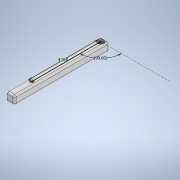
# Autodesk Inventor part: spincoater dispense arm
Saved by Autodesk Inventor 2020 (Build 240168000, 168)
## iProperties
Created: 2023-05-01
Part Number: spincoater dispense arm
Material: Generic
Document SubType Name: Modeling
Designer: Beaucage
Density: 1 g/cm^3
Appearance: Default
Author: Beaucage
Autodesk Inventor part; units mm, degrees
ref_plane "YZ Plane" through (0, 0, 0) normal (1, 0, 0) x (0, 1, 0)
ref_plane "XZ Plane" through (0, 0, 0) normal (0, 1, 0) x (-1, 0, 0)
ref_plane "XY Plane" through (0, 0, 0) normal (0, 0, 1) x (1, 0, 0)
sketch "Sketch1" plane through (0, 0, 0) normal (0, 1, 0) x (-1, 0, 0)
  line L0 (-6.35, 6.35) -> (6.35, 6.35)
  line L1 (6.35, 6.35) -> (6.35, -6.35)
  line L2 (6.35, -6.35) -> (-6.35, -6.35)
  line L3 (-6.35, -6.35) -> (-6.35, 6.35)
  line L4 (-6.35, 6.35) -> (6.35, -6.35) construction
  line L5 (6.35, 6.35) -> (-6.35, -6.35) construction
  circle A0 centre (0, 0) radius 4.7625
  dimension "d0" = 12.7
  dimension "d1" = 12.7
  dimension "d2" = 9.525
  constraints: 12 end point, 2 midpoint, 2 parallel, 1 centre point, 1 coincident, 1 horizontal, 1 perpendicular
  measures "d0" distance of L1.end L2.end
  measures "d1" distance of L0.end L1.end
  measures "d2" diameter of A0
extrude "Extrusion1" add sketch "Sketch1" along normal blind 12.7
sketch "Sketch2" plane through (-6.35, 0, 6.35) normal (0, 0, 1) x (1, 0, 0)
  line L0 (6.35, 0) -> (6.35, 6.35)
  circle A0 centre (6.35, 6.35) radius 1.5875
  dimension "d5" = 6.35
  dimension "d6" = 3.175
  constraints: 2 end point, 1 centre point, 1 coincident, 1 vertical
  measures "d5" distance of L0.start L0.end
  measures "d6" diameter of A0
extrude "Extrusion2" add sketch "Sketch2" against normal blind 4.445
sketch "Sketch3" plane through (-6.35, 0, 6.35) normal (0, 0, 1) x (1, 0, 0)
  line L0 (12.7, 0) -> (0, 0) projected
  line L1 (12.7, 0) -> (12.7, 12.7) projected
  line L2 (0, 0) -> (12.7, 0)
  line L3 (12.7, 0) -> (12.7, 12.7)
  line L4 (12.7, 12.7) -> (0, 12.7)
  line L5 (0, 12.7) -> (0, 0)
  point P0 (6.35, 0)
  constraints: 8 end point, 2 parallel, 1 horizontal, 1 perpendicular
extrude "Extrusion3" add sketch "Sketch3" along normal blind 127
fillet "Fillet1" radius 2.54 12 edges at (6.35, 12.7, 63.5) (6.35, 0, 63.5) (-6.35, 12.7, 63.5) (-6.35, 0, 63.5) (-6.35, 6.35, 133.35) (0, 0, 133.35) (6.35, 6.35, 133.35) (0, 12.7, 133.35) (-6.35, 6.35, -6.35) (6.35, 6.35, -6.35) (0, 12.7, -6.35) (0, 0, -6.35)
sketch "Sketch4" plane through (0, 12.7, 0) normal (0, 1, 0) x (1, 0, 0)
  line L0 (0, 0) -> (0, -101.854)
  line L1 (0, 0) -> (101.854, 0) construction
  dimension "d12" = 101.854
  dimension "d13" = 90
  constraints: 4 end point, 1 horizontal, 1 perpendicular, 1 vertical
  measures "d12" distance of L0.start L0.end
  measures "d13" angle of L0 L1
hole "Hole1" at (0, 12.7, 101.854) direction (0, -1, 0) diameter 5.4102 depth 6.35
hole "Hole2" at (0, 12.7, 101.854) direction (0, -1, 0) diameter 3.175 depth 25.4 tip angle 118
sketch "Sketch5" plane through (-6.35, 2.54, -3.81) normal (-1, 0, 0) x (0, 0, 1)
  line L0 (3.81, -2.54) -> (96.774, -2.54)
  line L1 (3.81, -2.54) -> (96.774, -2.54) construction
  line L2 (96.774, -2.54) -> (96.774, 3.81)
  line L3 (134.62, 0) -> (0, 0) projected
  line L4 (96.774, -2.54) -> (103.124, -2.54) construction
  point P0 (3.81, 10.16)
  dimension "d28" = 92.964
  dimension "d29" = 0
  dimension "d30" = 6.35
  dimension "d31" = 90
  constraints: 8 end point, 3 horizontal, 2 equal length, 1 perpendicular
  measures "d28" distance of L0.start L0.end
  measures "d29" distance between parallel lines of L0 L1
  measures "d30" distance of L1.end L2.end
  measures "d31" angle of L4 L2
hole "Hole3" at (-6.35, 6.35, 92.964) direction (1, 0, 0) diameter 5.4102 depth 6.35
body "Solid1"
